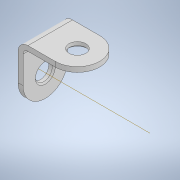
# Autodesk Inventor part: Angle Bracket
Saved by Autodesk Inventor 2022 (Build 260153000, 153)
## iProperties
Created: 2022-04-03
Part Number: Angle Bracket
Material: Generic
Document SubType Name: Modeling
Designer: Nick
Density: 1 g/cm^3
Appearance: Default
Author: Nick
Autodesk Inventor part; units mm, degrees
ref_plane "YZ Plane" through (0, 0, 0) normal (1, 0, 0) x (0, 1, 0)
ref_plane "XZ Plane" through (0, 0, 0) normal (0, 1, 0) x (-1, 0, 0)
sketch "Sketch1" plane through (0, 0, 0) normal (0, 0, 1) x (1, 0, 0)
  line L0 (0, 0) -> (0, 12)
  line L1 (0, 12) -> (12, 12)
  line L2 (12, 12) -> (12, 11)
  line L3 (12, 11) -> (1, 11)
  line L4 (1, 11) -> (1, 0)
  line L5 (1, 0) -> (0, 0)
  dimension "d0" = 12
  dimension "d1" = 12
  dimension "d2" = 1
  constraints: 12 end point, 2 horizontal, 2 perpendicular, 2 vertical, 1 parallel
  measures "d0" distance of L0.start L0.end
  measures "d1" distance of L0.end L1.end
  measures "d2" distance of L1.end L2.end
extrude "Extrusion1" add sketch "Sketch1" along normal blind 9
sketch "Sketch2" plane through (0, 0, 0) normal (-1, 0, 0) x (0, 0, 1)
  line L0 (9, 12) -> (9, 0) projected
  line L1 (0, 12) -> (9, 12) projected
  point P0 (0, 0)
  point P1 (4.5, 6)
  point P2 (9, 6)
  point P3 (4.5, 12)
  constraints: 2 midpoint, 1 horizontal alignment, 1 vertical alignment
sketch "Sketch5" plane through (1, 0, 0) normal (1, 0, 0) x (0, 0, -1)
  line L0 (0, 0) -> (0, 11) projected
  line L1 (0, 11) -> (-9, 11) projected
  line L2 (-9, 0) -> (-9, 11) projected
  line L3 (0, 0) -> (-9, 0) projected
  circle A0 centre (-4.5, 4.5) radius 4.5
  point P0 (0, 4.5)
  point P1 (-4.5, 0)
  point P2 (-9, 4.5)
  constraints: 3 tangent, 1 centre point
hole "Hole2" at (1, 4.5, 4.5) direction (-1, 0, 0) diameter 3.4 end through all countersink diameter 4 countersink angle 90 clearance for "Flat Head Machine Screw" size "M3" standard "Ansi Metric M Profile"
extrude "Extrusion3" cut sketch "Sketch5" against normal blind 16.002 contours L3 A0 L0 | L3 L2 A0
ref_plane "Work Plane1" through (1, 11, 0) normal (-0.7071, -0.7071, 0) x (0, 0, -1)
mirror "Mirror1" about plane through (1, 11, 0) normal (-0.7071, -0.7071, 0) of "Extrusion3", "Hole2"
fillet "Fillet1" radius 2 1 edges at (0, 12, 4.5)
fillet "Fillet2" radius 1 1 edges at (1, 11, 4.5)
equation "\"d1\" = d0"
body "Solid1"
